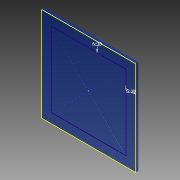
# Autodesk Inventor part: tray
Saved by Autodesk Inventor 2014 SP2 (Build 180246200, 246)
## iProperties
Created: 2016-04-26
Part Number: tray
Material: Generic
Document SubType Name: Modeling
Designer: cruiser
Density: 1 g/cm^3
Appearance: Clear - Blue
Author: cruiser
Autodesk Inventor part; units mm, degrees
ref_plane "YZ Plane" through (0, 0, 0) normal (1, 0, 0) x (0, 1, 0)
ref_plane "XZ Plane" through (0, 0, 0) normal (0, 1, 0) x (-1, 0, 0)
ref_plane "XY Plane" through (0, 0, 0) normal (0, 0, 1) x (1, 0, 0)
sketch "Sketch1" plane through (0, 0, 0) normal (0, 1, 0) x (-1, 0, 0)
  line L0 (97.325, -97.325) -> (-97.325, -97.325)
  line L1 (-97.325, -97.325) -> (-97.325, 97.325)
  line L2 (-97.325, 97.325) -> (97.325, 97.325)
  line L3 (97.325, 97.325) -> (97.325, -97.325)
  line L4 (97.325, -97.325) -> (-97.325, 97.325) construction
  line L5 (-97.325, -97.325) -> (97.325, 97.325) construction
  point P0 (0, 0)
  dimension "d0" = 194.65
  dimension "d1" = 194.65
  constraints: 12 end point, 2 midpoint, 2 parallel, 1 horizontal, 1 perpendicular
  measures "d0" distance of L1.end L2.end
  measures "d1" distance of L0.end L1.end
extrude "Extrusion1" add sketch "Sketch1" along normal blind 5.88
sketch "Sketch2" plane through (0, 5.88, 0) normal (0, 1, 0) x (1, 0, 0)
  circle A0 centre (-74.5, -74.5) radius 5
  line L0 (97.325, 97.325) -> (-97.325, 97.325) projected
  line L1 (-97.325, 97.325) -> (-97.325, -97.325) projected
  line L2 (80.5, -80.5) -> (-80.5, -80.5)
  line L3 (-80.5, -80.5) -> (-80.5, 80.5)
  line L4 (-80.5, 80.5) -> (80.5, 80.5)
  line L5 (80.5, 80.5) -> (80.5, -80.5)
  line L6 (80.5, -80.5) -> (-80.5, 80.5) construction
  line L7 (-80.5, -80.5) -> (80.5, 80.5) construction
  line L8 (75, -75) -> (-75, -75)
  line L9 (-75, -75) -> (-75, 75)
  line L10 (-75, 75) -> (75, 75)
  line L11 (75, 75) -> (75, -75)
  line L12 (75, -75) -> (-75, 75) construction
  line L13 (-75, -75) -> (75, 75) construction
  circle A1 centre (-74.5, -74.5) radius 6
  circle A2 centre (-88.9125, 62.75) radius 2.5
  line L14 (0, 0) -> (-75, 0)
  circle A3 centre (-88.9125, -62.75) radius 2.5
  circle A4 centre (-62.75, -88.9125) radius 2.5
  circle A5 centre (62.75, -88.9125) radius 2.5
  circle A6 centre (88.9125, -62.75) radius 2.5
  circle A7 centre (88.9125, 62.75) radius 2.5
  circle A8 centre (62.75, 88.9125) radius 2.5
  circle A9 centre (-62.75, 88.9125) radius 2.5
  dimension "d4" = 10
  dimension "d7" = 16.825
  dimension "d8" = 16.825
  dimension "d9" = 150
  dimension "d10" = 150
  dimension "d11" = 6
  dimension "d12" = 12
  dimension "d13" = 5
  dimension "d14" = 8.4125
  dimension "d15" = 62.75
  dimension "d18" = 360
  constraints: 26 end point, 10 centre point, 5 midpoint, 4 parallel, 2 horizontal, 2 perpendicular, 1 coincident, 1 point on line, 1 symmetric about line, 18 other
  measures "d4" diameter of A0
  measures "d7" distance between parallel lines of L0 L4
  measures "d8" distance between parallel lines of L1 L3
  measures "d9" distance of L9.end L10.end
  measures "d10" distance of L10.end L8.start
  measures "d11" distance from line of A0.centre L2
  measures "d12" diameter of A1
  measures "d13" diameter of A2
  measures "d14" distance from line of L3 A2.centre
  measures "d15" distance from line of A2.centre L14
extrude "Extrusion2" [suppressed]
sketch "Sketch4" plane through (0, 0, 0) normal (0, -1, 0) x (1, 0, 0)
  line L0 (-97.325, -97.325) -> (97.325, -97.325) projected
  line L1 (97.325, -97.325) -> (97.325, 97.325) projected
  line L2 (97.325, 97.325) -> (-97.325, 97.325) projected
  line L3 (-97.325, 97.325) -> (-97.325, -97.325) projected
  line L4 (-77.325, -77.325) -> (77.325, -77.325)
  line L5 (77.325, -77.325) -> (77.325, 77.325)
  line L6 (77.325, 77.325) -> (-77.325, 77.325)
  line L7 (-77.325, 77.325) -> (-77.325, -77.325)
  line L8 (-77.325, -77.325) -> (77.325, 77.325) construction
  line L9 (77.325, -77.325) -> (-77.325, 77.325) construction
  point P0 (0, 0)
  dimension "d20" = 20
  dimension "d21" = 20
  constraints: 12 end point, 2 midpoint, 2 parallel, 1 horizontal, 1 perpendicular
  measures "d20" distance between parallel lines of L1 L5
  measures "d21" distance between parallel lines of L2 L6
equation "\"d0\" = reservoir_x - 4 * sm_thickness"
equation "\"d1\" = reservoir_x - 4 * sm_thickness"
equation "\"d2\" = thick_acrylic"
equation "\"d4\" = stopper_diameter"
equation "\"d7\" = reservoir_overlap - 2 * sm_thickness"
equation "\"d8\" = reservoir_overlap - 2 * sm_thickness"
equation "\"d9\" = bed_x"
equation "\"d10\" = bed_y"
equation "\"d13\" = m5_diameter"
equation "\"d14\" = -sm_thickness + 0.5 * reservoir_overlap"
equation "\"d15\" = 0.25 * tray_y"
equation "\"d5\" = thick_acrylic"
equation "\"d20\" = reservoir_overlap"
equation "\"d21\" = reservoir_overlap"
equation "\"sm_thickness\" = 1.5875"
equation "\"thick_acrylic\" = 5.88"
equation "\"thin_acrylic\" = 3.15"
equation "\"clear_acrylic\" = 3.15"
equation "\"wood_thickness\" = 6.72"
equation "\"m3_diameter\" = 3"
equation "\"m4_diameter\" = 4"
equation "\"m5_diameter\" = 5"
equation "\"brass_insert_drill\" = 4"
equation "\"m5_brass_insert_drill\" = 6.7"
equation "\"m3_main_length\" = 14"
equation "\"m3_main_nut_width\" = 5.7"
equation "\"m3_main_nut_thickness\" = 2.5"
equation "\"m3_main_extra\" = 1"
equation "\"stepper_screw_space\" = 35"
equation "\"stepper_shaft_diameter\" = 5"
equation "\"stepper_body_diameter\" = 28"
equation "\"laser_body_diameter\" = 12"
equation "\"t_carrier\" = 5.88"
equation "\"t_wall\" = 5.88"
equation "\"t_window\" = 3.15"
equation "\"carrier_y\" = 251"
equation "\"carrier_z\" = 12"
equation "\"carrier_z2\" = 283.04"
equation "\"protection_slot\" = 36.2"
equation "\"protection_slot_offset\" = 45.25"
equation "\"window_z\" = 334.9125"
equation "\"window_y\" = 92.0625"
equation "\"window_slot\" = 25"
equation "\"door_sensor\" = 35"
equation "\"reservoir_x\" = 201"
equation "\"reservoir_y\" = 201"
equation "\"reservoir_overlap\" = 20"
equation "\"linear_bearing_spacing\" = 267"
equation "\"motor_spacing\" = 337"
equation "\"t_tray\" = 3.15"
equation "\"tray_border\" = 25"
equation "\"tray_x\" = 251"
equation "\"tray_y\" = 251"
equation "\"bed_x\" = 150"
equation "\"bed_y\" = 150"
equation "\"stopper_diameter\" = 10"
equation "\"brass_keep_out\" = 8"
equation "\"tape_keep_out\" = 2"
equation "\"tape_thickness\" = 2"
equation "\"t_crane\" = 6.72"
equation "\"end_stop_spacing\" = 19"
equation "\"thumb_nut_offset_y\" = 0"
equation "\"thumb_nut_diameter\" = 7"
equation "\"z_min_from_center\" = 115"
equation "\"t_frame\" = 6.72"
equation "\"frame_top_z\" = 386"
equation "\"frame_bottom_z\" = 275"
equation "\"frame_total_z\" = 661"
equation "\"frame_border\" = 46.35"
equation "\"frame_foot_z\" = 12"
equation "\"frame_tilt\" = 1deg"
equation "\"printer_z\" = 289"
equation "\"lcd_x\" = 72"
equation "\"lcd_y\" = 25"
equation "\"subframe_x\" = 195"
equation "\"subframe_y_offset\" = 27.5"
equation "\"laser_y_offset\" = 19.4"
equation "\"laser_diameter\" = 12"
equation "\"laser_z_offset\" = 55"
equation "\"laser_y\" = 35"
equation "\"laser_z\" = 18"
equation "\"laser_x\" = 24"
equation "\"t_galvo_frame\" = 6.72"
equation "\"galvo_frame_x\" = 66"
equation "\"galvo_frame_z\" = 65"
equation "\"galvo_frame_y_offset\" = 27.5"
equation "\"drawer_x\" = 257.3"
equation "\"drawer_y\" = 88.65"
equation "\"drawer_z\" = 278.175"
equation "\"drawer_z_from_bottom\" = 25"
equation "\"crane_z2\" = 12"
equation "\"bed_z\" = 25.4"
equation "\"nema17_x\" = 43"
equation "\"bed_z2\" = 79.6"
equation "\"very_thick_acrylic\" = 9.45"
equation "\"m5_press_nut_drill\" = 6.5"
equation "\"visor_x\" = 257.3"
equation "\"m3_press_nut_drill\" = 4.5"
equation "\"window_overlap\" = 47.4675"
equation "\"visor_y\" = 110.2375"
equation "\"door_overlap\" = 47.4675"
equation "\"door_z\" = 334.9125"
equation "\"acrylic_into_frame\" = 5"
equation "\"m3_head\" = 6"
equation "\"door_x\" = 251"
equation "\"drawer_support_from_top\" = 47.4675"
body "Solid1"
